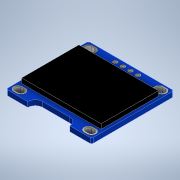
# Autodesk Inventor part: SSD1306
Saved by Autodesk Inventor 2021 (Build 250183000, 183)
## iProperties
Created: 2021-07-21
Part Number: SSD1306
Material: Generic
Document SubType Name: Modeling
Designer: ermoz
Density: 1 g/cm^3
Appearance: Default
Author: ermoz
Autodesk Inventor part; units mm, degrees
ref_plane "YZ Plane" through (0, 0, 0) normal (1, 0, 0) x (0, 1, 0)
ref_plane "XZ Plane" through (0, 0, 0) normal (0, 1, 0) x (-1, 0, 0)
ref_plane "XY Plane" through (0, 0, 0) normal (0, 0, 1) x (1, 0, 0)
sketch "Sketch1" plane through (0, 0, 0) normal (0, 1, 0) x (-1, 0, 0)
  line L0 (14.2292, 13.75) -> (14.2708, -13.75)
  line L1 (14.2708, -13.75) -> (-14.2292, -13.75)
  line L2 (-14.2292, -13.75) -> (-14.2708, 13.75)
  line L3 (-14.2708, 13.75) -> (14.2708, -13.75) construction
  line L4 (14.2292, 13.75) -> (-14.2292, -13.75) construction
  line L5 (14.2292, 13.75) -> (7, 13.75)
  line L6 (4.5, 11.25) -> (-4.5, 11.25)
  line L7 (-7, 13.75) -> (-14.2708, 13.75)
  arc A0 (-7, 13.75) -> (-4.5, 11.25) centre (-4.5, 13.75) ccw
  arc A1 (4.5, 11.25) -> (7, 13.75) centre (4.5, 13.75) ccw
  line L8 (0, 0) -> (0, -4.4345)
  line L9 (0, 11.25) -> (0, 7.5255)
  dimension "d0" = 28.5
  dimension "d1" = 27.5
  dimension "d2" = 2.5
  dimension "d3" = 14
  constraints: 22 end point, 4 point on circle, 3 midpoint, 2 centre point, 2 collinear, 2 horizontal, 2 parallel, 2 point on line, 2 tangent, 2 vertical, 1 line through centre
  measures "d0" distance of L0.end L1.end
  measures "d1" distance of L0.start L0.end
  measures "d2" distance between parallel lines of L7 L6
  measures "d3" distance of L7.start L5.end
extrude "Extrusion1" add sketch "Sketch1" along normal blind 1.7
chamfer "Chamfer1" distance 0.5 angle 45 4 edges at (14.2708, 0.85, 13.75) (-14.2292, 0.85, 13.75) (14.2292, 0.85, -13.75) (-14.2708, 0.85, -13.75)
sketch "Sketch2" plane through (0, 1.7, 0) normal (0, 1, 0) x (1, 0, 0)
  line L0 (-13.2678, 11.75) -> (-10.2678, 11.75) construction
  line L1 (-12.2678, 10.75) -> (-11.2678, 10.75)
  line L2 (-11.2678, 12.75) -> (-12.2678, 12.75)
  arc A0 (-12.2678, 12.75) -> (-12.2678, 10.75) centre (-12.2678, 11.75) ccw
  arc A1 (-11.2678, 10.75) -> (-11.2678, 12.75) centre (-11.2678, 11.75) ccw
  line L3 (-11.2678, 13.25) -> (-12.2678, 13.25)
  arc A2 (-12.2678, 13.25) -> (-12.2678, 10.25) centre (-12.2678, 11.75) ccw
  line L4 (-12.2678, 10.25) -> (-11.2678, 10.25)
  arc A3 (-11.2678, 10.25) -> (-11.2678, 13.25) centre (-11.2678, 11.75) ccw
  line L5 (13.7292, 13.75) -> (-13.7708, 13.75) projected
  line L6 (-14.2701, 13.25) -> (-14.2299, -13.25) projected
  line L7 (0, 0) -> (-2.3297, 0)
  line L8 (0, 0) -> (0, 4.8141)
  line L9 (13.2678, 11.75) -> (10.2678, 11.75) construction
  line L10 (12.2678, 10.75) -> (11.2678, 10.75)
  line L11 (11.2678, 12.75) -> (12.2678, 12.75)
  arc A4 (12.2678, 10.75) -> (12.2678, 12.75) centre (12.2678, 11.75) ccw
  arc A5 (11.2678, 12.75) -> (11.2678, 10.75) centre (11.2678, 11.75) ccw
  line L12 (11.2678, 13.25) -> (12.2678, 13.25)
  arc A6 (12.2678, 10.25) -> (12.2678, 13.25) centre (12.2678, 11.75) ccw
  line L13 (12.2678, 10.25) -> (11.2678, 10.25)
  arc A7 (11.2678, 13.25) -> (11.2678, 10.25) centre (11.2678, 11.75) ccw
  line L14 (-13.2678, -11.75) -> (-10.2678, -11.75) construction
  line L15 (-12.2678, -10.75) -> (-11.2678, -10.75)
  line L16 (-11.2678, -12.75) -> (-12.2678, -12.75)
  arc A8 (-12.2678, -10.75) -> (-12.2678, -12.75) centre (-12.2678, -11.75) ccw
  arc A9 (-11.2678, -12.75) -> (-11.2678, -10.75) centre (-11.2678, -11.75) ccw
  line L17 (-11.2678, -13.25) -> (-12.2678, -13.25)
  arc A10 (-12.2678, -10.25) -> (-12.2678, -13.25) centre (-12.2678, -11.75) ccw
  line L18 (-12.2678, -10.25) -> (-11.2678, -10.25)
  arc A11 (-11.2678, -13.25) -> (-11.2678, -10.25) centre (-11.2678, -11.75) ccw
  line L19 (12.2678, -10.25) -> (11.2678, -10.25)
  line L20 (12.2678, -10.75) -> (11.2678, -10.75)
  line L21 (11.2678, -12.75) -> (12.2678, -12.75)
  arc A12 (12.2678, -12.75) -> (12.2678, -10.75) centre (12.2678, -11.75) ccw
  arc A13 (11.2678, -10.75) -> (11.2678, -12.75) centre (11.2678, -11.75) ccw
  arc A14 (11.2678, -10.25) -> (11.2678, -13.25) centre (11.2678, -11.75) ccw
  arc A15 (12.2678, -13.25) -> (12.2678, -10.25) centre (12.2678, -11.75) ccw
  line L22 (11.2678, -13.25) -> (12.2678, -13.25)
  line L23 (13.2678, -11.75) -> (10.2678, -11.75) construction
  circle A16 centre (-3.81, 12.25) radius 0.75
  circle A17 centre (-1.27, 12.25) radius 0.75
  circle A18 centre (1.27, 12.25) radius 0.75
  circle A19 centre (3.81, 12.25) radius 0.75
  circle A20 centre (-3.81, 12.25) radius 0.425
  circle A21 centre (-1.27, 12.25) radius 0.425
  circle A22 centre (1.27, 12.25) radius 0.425
  circle A23 centre (3.81, 12.25) radius 0.425
  point P0 (-11.7678, 11.75)
  point P1 (11.7678, 11.75)
  point P2 (-11.7678, -11.75)
  point P3 (11.7678, -11.75)
  dimension "d9" = 3
  dimension "d10" = 2
  dimension "d11" = 0.5
  dimension "d12" = 0.5
  dimension "d13" = 2
  dimension "d22" = 2.54
  dimension "d23" = 2.54
  dimension "d24" = 2.54
  dimension "d25" = 1.5
  dimension "d26" = 0.85
  dimension "d27" = 1.5
  constraints: 52 end point, 40 point on circle, 40 symmetric about line, 24 centre point, 8 point on line, 6 equal radius, 4 coincident, 4 tangent, 2 horizontal, 2 horizontal alignment, 2 parallel, 1 midpoint, 1 vertical, 15 other
  measures "d9" distance of L0.start L0.end
  measures "d10" diameter of A1
  measures "d11" radial gap between concentric circles of A1 A3
  measures "d12" distance between parallel lines of L5 L3
  measures "d13" distance from line of L6 A0.centre
  measures "d22" distance of A16.centre A17.centre
  measures "d23" distance of A17.centre A18.centre
  measures "d24" distance of A18.centre A19.centre
  measures "d25" diameter of A16
  measures "d26" diameter of A23
  measures "d27" distance from line of L5 A19.centre
extrude "Extrusion2" cut sketch "Sketch2" against normal through all contours A0 L2 A1 L1 | A3 L4 A2 L3 | L10 A5 L11 A4 | L12 A6 L13 A7 | L15 A9 L16 A8 | L17 A10 L18 A11 | A15 L22 A14 L19 | A12 L21 A13 L20 | A16 | A17 | A18 | A19 | A20 | A21 | A22 | A23
extrude "Extrusion3" add sketch "Sketch2" against normal up to surface (1.7 mm away) separate body
sketch "Sketch3" plane through (0, 1.7, 0) normal (0, 1, 0) x (1, 0, 0)
  line L0 (-13.25, 9.55) -> (13.25, 9.55)
  line L1 (13.25, 9.55) -> (13.25, -9.55)
  line L2 (13.25, -9.55) -> (-13.25, -9.55)
  line L3 (-13.25, -9.55) -> (-13.25, 9.55)
  line L4 (-13.25, 9.55) -> (13.25, -9.55) construction
  line L5 (13.25, 9.55) -> (-13.25, -9.55) construction
  point P0 (0, 0)
  point P1 (0, 0)
  point P2 (0, 0)
  point P3 (0, 0)
  dimension "d18" = 19.1
  dimension "d19" = 26.5
  constraints: 12 end point, 4 midpoint, 2 coincident, 2 parallel, 1 horizontal, 1 perpendicular
  measures "d18" distance of L0.end L1.end
  measures "d19" distance of L0.start L0.end
extrude "Extrusion4" add sketch "Sketch3" along normal blind 1.6 separate body
body "Solid1"
body "Solid2"
body "Solid3"
